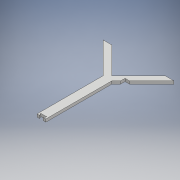
# Autodesk Inventor part: Liu_Inital_Y
Saved by Autodesk Inventor 2017 (Build 210142000, 142)
## iProperties
Created: 2016-09-23
Part Number: Liu_Inital_Y
Material: Generic
Document SubType Name: Modeling
Designer: jliu
Density: 1 g/cm^3
Appearance: Default
Mass: 4.46188 g
Surface Area: 40.1011 cm^2
Volume: 4.46188 cm^3
Author: jliu
Autodesk Inventor part; units mm, degrees
ref_plane "YZ Plane" through (0, 0, 0) normal (1, 0, 0) x (0, 1, 0)
ref_plane "XZ Plane" through (0, 0, 0) normal (0, 1, 0) x (-1, 0, 0)
ref_plane "XY Plane" through (0, 0, 0) normal (0, 0, 1) x (1, 0, 0)
sketch "Sketch1" plane through (0, 0, 0) normal (0, 0, 1) x (1, 0, 0)
  line L0 (5, 0) -> (5, 75)
  line L1 (5, 75) -> (0, 75) construction
  line L2 (5, 75) -> (55, 75) construction
  line L3 (40.3553, 110.3553) -> (30.3553, 110.3553)
  line L4 (30.3553, 110.3553) -> (0, 80)
  line L5 (0, 0) -> (0, 80) construction
  line L6 (5, 0) -> (2, 0)
  line L7 (2, 0) -> (3.5, 2.5981)
  line L8 (3.5, 2.5981) -> (0, 2.5981)
  line L9 (-5, 0) -> (-5, 75)
  line L10 (-5, 75) -> (-40.3553, 110.3553)
  line L11 (-40.3553, 110.3553) -> (-30.3553, 110.3553)
  line L12 (-30.3553, 110.3553) -> (0, 80)
  line L13 (-5, 0) -> (-2, 0)
  line L14 (-2, 0) -> (-3.5, 2.5981)
  line L15 (-3.5, 2.5981) -> (0, 2.5981)
  line L16 (10, 80) -> (10, 85)
  line L17 (10, 85) -> (15, 85)
  line L18 (5, 75) -> (10, 80)
  line L19 (15, 85) -> (40.3553, 110.3553)
  dimension "d0" = 5
  dimension "d1" = 75
  dimension "d2" = 50
  dimension "d5" = 10
  dimension "d6" = 3
  dimension "d7" = 3
  dimension "d8" = 60
  dimension "d9" = 5
  dimension "d15" = 45
  dimension "d16" = 5
  dimension "d17" = 5
  constraints: 40 end point, 6 symmetric about line, 3 horizontal, 3 perpendicular, 2 collinear, 2 parallel, 2 vertical, 1 point on line
  measures "d0" distance of L5.start L0.start
  measures "d1" distance of L0.start L0.end
  measures "d2" distance of L0.end L3.start
  measures "d5" distance of L3.start L3.end
  measures "d6" distance of L0.start L6.end
  measures "d7" distance of L6.end L7.end
  measures "d8" angle of L6 L7
  measures "d9" distance between parallel lines of L5 L0
  measures "d15" angle of L18 L2
  measures "d16" distance from line of L2 L16.start
  measures "d17" distance of L17.end L16.end
extrude "Extrusion1" add sketch "Sketch1" along normal mid plane 3.175
body "Solid1"
